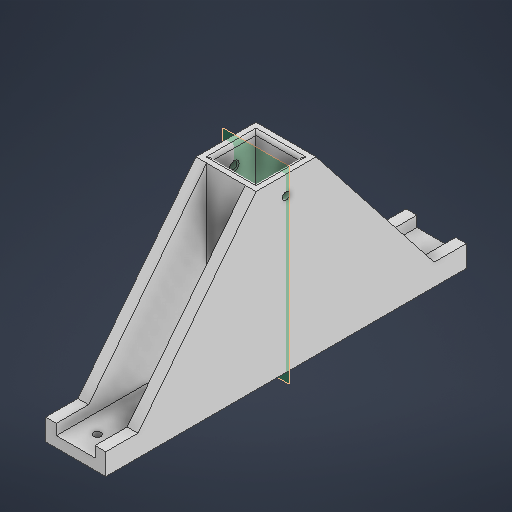
# Autodesk Inventor part: SoportePrincipal
Saved by Autodesk Inventor 2026.1 (Build 301233020, 233B)
## iProperties
Created: 2025-10-19
Part Number: SoportePrincipal
Material: Generic
Document SubType Name: Modeling
Designer: tito.luyo
Density: 1 g/cm^3
Appearance: Default
Author: tito.luyo
Autodesk Inventor part; units mm, degrees
ref_plane "YZ Plane" through (0, 0, 0) normal (1, 0, 0) x (0, 1, 0)
ref_plane "XZ Plane" through (0, 0, 0) normal (0, 1, 0) x (-1, 0, 0)
sketch "Sketch1" plane through (0, 0, 0) normal (0, 1, 0) x (-1, 0, 0)
  line L0 (0, 0) -> (28, 0)
  line L1 (28, 0) -> (28, -28)
  line L2 (28, -28) -> (0, -28)
  line L3 (0, -28) -> (0, 0)
  line L4 (24.125, -3.875) -> (3.875, -3.875)
  line L5 (3.875, -3.875) -> (3.875, -24.125)
  line L6 (3.875, -24.125) -> (24.125, -24.125)
  line L7 (24.125, -24.125) -> (24.125, -3.875)
  line L8 (24.125, -3.875) -> (3.875, -24.125) construction
  line L9 (3.875, -3.875) -> (24.125, -24.125) construction
  line L10 (0, 0) -> (28, -28) construction
  line L11 (28, 0) -> (0, -28) construction
  point P0 (14, -14)
  dimension "externo" = 28
  dimension "externo2" = 28
  dimension "interno" = 20.25
  dimension "interno2" = 20.25
  constraints: 24 end point, 4 parallel, 3 midpoint, 2 horizontal, 2 perpendicular
  measures "externo" distance of L1.end L2.end
  measures "externo2" distance of L0.end L1.end
  measures "interno" distance of L6.end L5.end
  measures "interno2" distance of L5.end L4.end
extrude "principal" add sketch "Sketch1" along normal blind 80
sketch "Sketch2" plane through (-28, 80, -28) normal (-1, 0, 0) x (0, 0, 1)
  circle A0 centre (14, -8.7403) radius 1.75
  point P0 (28, -80)
  dimension "hueco_tornillo" = 3.5
  constraints: 1 centre point
  measures "hueco_tornillo" diameter of A0
extrude "hueco1" cut sketch "Sketch2" against normal blind 7.75
sketch "Sketch3" plane through (0, 80, 0) normal (1, 0, 0) x (0, 0, -1)
  circle A0 centre (14, -8.7403) radius 1.75 projected
  circle A1 centre (14, -8.7403) radius 1.75
  point P0 (0, -80)
  dimension "hueco_tornillo_2" = 3.5
  constraints: 1 centre point, 1 coincident
  measures "hueco_tornillo_2" diameter of A1
extrude "hueco2" cut sketch "Sketch3" against normal blind 7.75
fillet "hueco_Fillet" radius 0.5 2 edges at (-3.875, 71.2597, -12.25) (-24.125, 71.2597, -15.75)
sketch "Sketch4" plane through (0, 0, -28) normal (0, 0, -1) x (-1, 0, 0)
  line L0 (28, 0) -> (0, 0) projected
  line L1 (0, 0) -> (28, 0)
  line L2 (28, 0) -> (28, 5)
  line L3 (28, 5) -> (0, 5)
  line L4 (0, 5) -> (0, 0)
  line L5 (0, 5) -> (5, 5)
  line L6 (5, 5) -> (5, 10)
  line L7 (5, 10) -> (0, 10)
  line L8 (0, 10) -> (0, 5)
  line L9 (28, 5) -> (23, 5)
  line L10 (23, 5) -> (23, 10)
  line L11 (23, 10) -> (28, 10)
  line L12 (28, 10) -> (28, 5)
  point P0 (23, 5)
  point P1 (5, 5)
  dimension "lateral_ancho" = 28
  dimension "lateral_espesor" = 5
  dimension "lateral_refuerzo_1_ancho" = 5
  dimension "lateral_refuerzo_1_alto" = 5
  dimension "lateral_refuerzo_2_ancho" = 5
  dimension "lateral_refuerzo_2_alto" = 5
  constraints: 24 end point, 6 parallel, 3 horizontal, 3 perpendicular
  measures "lateral_ancho" distance of L3.end L2.end
  measures "lateral_espesor" distance of L2.end L1.end
  measures "lateral_refuerzo_1_ancho" distance of L7.end L6.end
  measures "lateral_refuerzo_1_alto" distance of L6.end L5.end
  measures "lateral_refuerzo_2_ancho" distance of L10.end L11.end
  measures "lateral_refuerzo_2_alto" distance of L9.end L10.end
extrude "lateral" add sketch "Sketch4" along normal blind 70
sketch "Sketch5" plane through (0, 0, 0) normal (1, 0, 0) x (0, 0, -1)
  line L0 (0, 80) -> (28, 80) projected
  line L1 (28, 10) -> (28, 80) projected
  line L2 (28, 80) -> (28, 10)
  line L3 (28, 10) -> (83, 10)
  line L4 (83, 10) -> (28, 80)
  point P0 (0, 0)
  dimension "refuerzo" = 55
  constraints: 6 end point, 1 perpendicular, 1 vertical
  measures "refuerzo" distance of L1.start L3.end
extrude "escuadra" add sketch "Sketch5" against normal blind 5
ref_plane "Work Plane1" through (-14, 0, 0) normal (1, 0, 0) x (0, 0, -1)
mirror "escuadra_Mirror" about plane through (-14, 0, 0) normal (1, 0, 0) of "escuadra"
sketch "Sketch6" plane through (-23, 5, -28) normal (0, 1, 0) x (1, 0, 0)
  circle A0 centre (9, 60) radius 1.75
  line L0 (0, 70) -> (18, 70) projected
  point P0 (23, -28)
  dimension "hueco_tornillo_lateral" = 3.5
  dimension "hueco_lateral_sep" = 10
  constraints: 1 centre point
  measures "hueco_tornillo_lateral" diameter of A0
  measures "hueco_lateral_sep" distance from line of L0 A0.centre
extrude "hueco_lateral" cut sketch "Sketch6" against normal blind 5
ref_plane "Work Plane2" through (-5, 5, -14) normal (0, 0, -1) x (-1, 0, 0)
mirror "lateral_mirror" about plane through (-5, 5, -14) normal (0, 0, -1) of "escuadra", "escuadra_Mirror", "lateral", "hueco_lateral"
fillet "entrada_Fillet" radius 1.5 4 edges at (-24.125, 80, -14) (-14, 80, -3.875) (-3.875, 80, -14) (-14, 80, -24.125)
equation "\"externo2\" = externo"
equation "\"interno2\" = interno"
equation "\"hueco_profundidad\" = externo - interno"
equation "\"hueco_tornillo_2\" = hueco_tornillo"
equation "\"hueco_profundidad_2\" = hueco_profundidad"
equation "\"lateral_ancho\" = externo"
equation "\"lateral_refuerzo_1_ancho\" = lateral_espesor"
equation "\"lateral_refuerzo_1_alto\" = lateral_espesor"
equation "\"lateral_refuerzo_2_ancho\" = lateral_espesor"
equation "\"lateral_refuerzo_2_alto\" = lateral_espesor"
equation "\"d23\" = lateral_espesor"
equation "\"hueco_tornillo_lateral\" = hueco_tornillo"
equation "\"d27\" = lateral_espesor"
body "Solid1"
